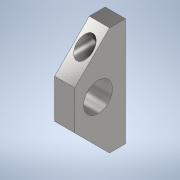
# Autodesk Inventor part: Glidelejrehus
Saved by Autodesk Inventor 2022.2 (Build 262287010, 287A)
## iProperties
Created: 2022-04-19
Part Number: Glidelejrehus
Material: Steel, Galvanized
Document SubType Name: Modeling
Designer: Finn Oriwohl
Density: 7.85 g/cm^3
Appearance: Galvanized
Author: Finn Oriwohl
Autodesk Inventor part; units mm, degrees
ref_plane "YZ Plane" through (0, 0, 0) normal (1, 0, 0) x (0, 1, 0)
ref_plane "XZ Plane" through (0, 0, 0) normal (0, 1, 0) x (-1, 0, 0)
ref_plane "XY Plane" through (0, 0, 0) normal (0, 0, 1) x (1, 0, 0)
sketch "Sketch1" plane through (0, 0, 0) normal (0, 0, 1) x (1, 0, 0)
  point P0 (0, 0)
sketch "Sketch2" plane through (0, 0, 0) normal (1, 0, 0) x (0, 1, 0)
  line L0 (13.1468, 0) -> (76.0129, 0) projected
  line L1 (13.1468, 0) -> (88.1468, 0)
  circle A0 centre (50.6468, 19) radius 10
  line L2 (13.1468, 35) -> (88.1468, 35)
  line L3 (13.1468, 0) -> (13.1468, 35)
  line L4 (88.1468, 0) -> (88.1468, 35)
  point P0 (0, 0)
  point P1 (90.0129, 0)
  dimension "d0" = 75
  dimension "d1" = 20
  dimension "d3" = 16
  dimension "d5" = 35
  dimension "d8" = 37.5
  constraints: 8 end point, 2 horizontal, 2 perpendicular, 1 centre point, 1 other
  measures "d0" distance of L0.start L1.end
  measures "d1" diameter of A0
  measures "d3" distance from line of L2 A0.centre
  measures "d5" distance of L1.end L2.end
  measures "d8" distance from line of L4 A0.centre
extrude "Extrusion1" add sketch "Sketch2" against normal blind 14
sketch "Sketch3" plane through (0, 13.1468, 35) normal (0, 0, 1) x (1, 0, 0)
  line L0 (0, 75) -> (0, 0) projected
  line L1 (0, 75) -> (-14, 75) projected
  line L2 (-14, 0) -> (-14, 75) projected
  line L3 (0, 0) -> (-14, 0) projected
  line L4 (0, 75) -> (0, 0) projected
  line L5 (0, 37.5) -> (-14, 37.5)
  point P0 (0, -13.1468)
  point P1 (-7, 10)
  point P2 (-7, 65)
  dimension "d12" = 7
  dimension "d13" = 14
  dimension "d14" = 10
  constraints: 2 end point, 2 midpoint, 1 symmetric about line
  measures "d12" distance from line of L0 point (-7, 10)
  measures "d13" distance of L0.end L2.start
  measures "d14" distance from line of point (-7, 10) L3
hole "Hole1" at (-7, 23.1468, 35) at (-7, 78.1468, 35) direction (0, 0, -1) diameter 6.6 end through all counterbore diameter 11 counterbore depth 25 clearance for "Socket Head Cap Screw ISO 4762" size "M6" standard "ISO"
chamfer "Chamfer1" distance 24 angle 45 2 edges at (-7, 13.1468, 35) (-7, 88.1468, 35)
equation "\"d8\" = 0.5 * d0"
equation "\"d12\" = 0.5 * d13"
body "Solid1"
